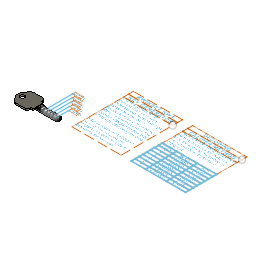
KWIKSET+KW1+KEYGEN (Autodesk Fusion 360 design; units mm, degrees)
Autodesk Fusion 360 part; units mm, degrees
note: some values were not read from the file. Set by a fixed rule: which sketch regions a step uses.
sketch "Sketch1" plane through (0, 0, 0) normal (0, 0, 1) x (1, 0, 0)
  line L0 (0, 0) -> (27.94, 0) construction
  line L1 (0, -4.2418) -> (27.94, -4.2418)
  line L2 (0, 4.2418) -> (27.94, 4.2418)
  line L3 (-3, -6.4) -> (0, -6.4)
  line L4 (0, 6.4) -> (-3, 6.4)
  line L5 (-18.6, 11) -> (-3, 11)
  line L6 (-3, -11) -> (-18.6, -11)
  line L7 (-25, -3.3728) -> (-25, 3.3728)
  line L8 (-18.6, 11) -> (-25, 3.3728)
  line L9 (-25, 11) -> (-33.2141, 11) construction
  line L10 (-18.6, -11) -> (-25, -3.3728)
  line L11 (-18.6, -11) -> (-34.3032, -11) construction
  line L12 (-3, 11) -> (-3, 6.4)
  line L13 (-3, -6.4) -> (-3, -11)
  arc A0 (-3, 8.5) -> (-5.5, 11) centre (-5.5, 8.5) ccw
  arc A1 (-5.5, -11) -> (-3, -8.5) centre (-5.5, -8.5) ccw
  line L14 (27.94, 4.2418) -> (27.94, -4.2418)
  line L15 (23.2107, 4.2418) -> (27.6471, -0.1946)
  line L16 (23.2107, 4.2418) -> (33.0981, 4.2418) construction
  line L17 (0, -0.9017) -> (27.94, -0.9017) construction
  line L18 (25.0141, -4.2418) -> (27.6471, -1.6088)
  line L19 (25.0141, -4.2418) -> (38.1109, -4.2418) construction
  arc A2 (27.6471, -1.6088) -> (27.3724, 0) centre (26.94, -0.9017) ccw
  line L20 (0, 4.2418) -> (0, 6.4)
  line L21 (0, -6.4) -> (0, -4.2418)
  dimension "d6" = 27.94
  dimension "d7" = 4.2418
  dimension "d8" = -4.2418
  dimension "d10" = 6.4
  dimension "d11" = 6.4
  dimension "d13" = 3
  dimension "d14" = 11
  dimension "d15" = 11
  dimension "d17" = 50
  dimension "d19" = 50
  dimension "d21" = 6.4
  dimension "d23" = 5
  dimension "d24" = 5
  dimension "d25" = 22
  dimension "d26" = 7.6272
  dimension "d27" = 7.6272
  dimension "d29" = 45
  dimension "d30" = 3.3401
  dimension "d31" = 2
  dimension "d32" = 45
  constraint coincident L0.start origin
  constraint horizontal L0
  constraint horizontal L3
  constraint vertical L21
  constraint horizontal L4
  constraint coincident L0.start L21
  constraint horizontal L5
  constraint vertical L12
  constraint horizontal L6
  constraint vertical L7
  constraint horizontal L9
  constraint horizontal L11
  constraint tangent L5 A0
  constraint tangent L12 A0
  constraint tangent L6 A1
  constraint tangent L12 A1
  constraint collinear L12 L13
  constraint coincident L5 A0.end
  constraint coincident L12 A0.start
  constraint coincident L13 A1.end
  constraint coincident L6 A1.start
  constraint perpendicular L1 L14
  constraint horizontal L16
  constraint coincident L2 L15.start
  constraint coincident L17.start L21
  constraint coincident L14 L17.end
  constraint perpendicular L14 L17
  constraint coincident L17 A2.centre
  constraint tangent L14 A2
  constraint horizontal L19
  constraint coincident L1 L18.start
  constraint coincident L0.end L14
  constraint tangent L18 A2
  constraint tangent L15 A2
  constraint coincident L0 A2.end
  constraint coincident A2 L15.end
  constraint collinear L20 L21
  measures "d6" distance of L0.start L0.end
  measures "d10" distance of L0 L4
  measures "d11" distance of L0 L3
  measures "d13" distance of L12 L21
  measures "d14" distance of L0 L5
  measures "d15" distance of L0 L6
  measures "d17" angle of L8 L9
  measures "d19" angle of L10 L11
  measures "d21" distance of L9.start L5.start
  measures "d23" diameter of A0
  measures "d24" diameter of A1
  measures "d25" distance of L7 L12
  measures "d26" vertical distance of L5.start L7.end
  measures "d27" vertical distance of L6.end L7.start
  measures "d29" angle of L15 L16
  measures "d30" distance of L1 L17
  measures "d31" diameter of A2
  measures "d32" angle of L18 L19
extrude "Extrude1" add sketch "Sketch1" along normal blind 2 contours L1 L2 L3 L4 L5 L6 L7 L8 L10 L12 L13 A0 A1 L15 L18 A2 L20 L21
fillet "Fillet1" radius 1 2 edges at (0, -6.4, 1) (0, 6.4, 1)
fillet "Fillet1" radius 4 4 edges at (-18.6, -11, 1) (-25, -3.3728, 1) (-25, 3.3728, 1) (-18.6, 11, 1)
sketch "Sketch2" plane through (0, 0, 2) normal (0, 0, 1) x (-1, 0, 0)
  line L0 (3, 6.4) -> (1, 6.4)
  line L1 (0, 5.4) -> (0, 4.2418)
  line L2 (0, 4.2418) -> (-25.0141, 4.2418)
  line L3 (-25.0141, 4.2418) -> (-27.6471, 1.6088)
  arc A0 (-27.6471, 1.6088) -> (-27.6471, 0.1946) centre (-26.94, 0.9017) ccw
  line L4 (-27.6471, 0.1946) -> (-23.2107, -4.2418)
  line L5 (-23.2107, -4.2418) -> (0, -4.2418)
  line L6 (0, -4.2418) -> (0, -5.4)
  line L7 (1, -6.4) -> (3, -6.4)
  line L8 (3, -6.4) -> (3, -8.5)
  arc A1 (3, -8.5) -> (5.5, -11) centre (5.5, -8.5) ccw
  line L9 (5.5, -11) -> (16.7348, -11)
  line L10 (19.7989, -9.5712) -> (24.0642, -4.488)
  line L11 (25, -1.9169) -> (25, 1.9169)
  line L12 (24.0642, 4.488) -> (19.7989, 9.5712)
  line L13 (16.7348, 11) -> (5.5, 11)
  arc A2 (5.5, 11) -> (3, 8.5) centre (5.5, 8.5) ccw
  line L14 (3, 8.5) -> (3, 6.4)
  line L15 (0, 4.2418) -> (0, -4.2418) construction
  line L16 (-6.2738, -4.2418) -> (-6.2738, 4.2418) construction
  line L17 (-10.0838, -4.2418) -> (-10.0838, 4.2418) construction
  line L18 (-13.8938, -4.2418) -> (-13.8938, 4.2418) construction
  line L19 (-17.7038, -4.2418) -> (-17.7038, 4.2418) construction
  line L20 (-21.5138, -4.2418) -> (-21.5138, 4.2418) construction
  line L21 (-5.207, -4.2418) -> (-5.207, 4.2418) construction
  line L22 (-7.3406, -4.2418) -> (-7.3406, 4.2418) construction
  line L23 (-9.017, -4.2418) -> (-9.017, 4.2418) construction
  line L24 (-11.1506, -4.2418) -> (-11.1506, 4.2418) construction
  line L25 (-12.827, -4.2418) -> (-12.827, 4.2418) construction
  line L26 (-14.9606, -4.2418) -> (-14.9606, 4.2418) construction
  line L27 (-16.637, -4.2418) -> (-16.637, 4.2418) construction
  line L28 (-18.7706, -4.2418) -> (-18.7706, 4.2418) construction
  line L29 (-20.447, -4.2418) -> (-20.447, 4.2418) construction
  line L30 (-22.5806, -4.2418) -> (-22.5806, 4.2418) construction
  line L31 (-5.207, -3.5306) -> (-7.3406, -3.5306)
  line L32 (-9.017, -1.778) -> (-11.1506, -1.778)
  line L33 (-12.827, -2.9464) -> (-14.9606, -2.9464)
  line L34 (-16.637, -3.5306) -> (-18.7706, -3.5306)
  line L35 (-20.447, -1.778) -> (-22.5806, -1.778)
  line L36 (-5.207, -3.5306) -> (-0.9644, -7.7732)
  line L37 (-5.207, -3.5306) -> (0.793, -3.5306) construction
  line L38 (-7.3406, -3.5306) -> (-11.5832, -7.7732)
  line L39 (-7.3406, -3.5306) -> (-13.3406, -3.5306) construction
  line L40 (-9.017, -1.778) -> (-4.7744, -6.0206)
  line L41 (-9.017, -1.778) -> (-3.017, -1.778) construction
  line L42 (-11.1506, -1.778) -> (-15.3932, -6.0206)
  line L43 (-11.1506, -1.778) -> (-17.1506, -1.778) construction
  line L44 (-12.827, -2.9464) -> (-8.5844, -7.189)
  line L45 (-12.827, -2.9464) -> (-6.827, -2.9464) construction
  line L46 (-14.9606, -2.9464) -> (-19.2032, -7.189)
  line L47 (-14.9606, -2.9464) -> (-20.9606, -2.9464) construction
  line L48 (-16.637, -3.5306) -> (-12.3944, -7.7732)
  line L49 (-16.637, -3.5306) -> (-10.637, -3.5306) construction
  line L50 (-18.7706, -3.5306) -> (-23.0132, -7.7732)
  line L51 (-18.7706, -3.5306) -> (-24.7706, -3.5306) construction
  line L52 (-20.447, -1.778) -> (-16.2044, -6.0206)
  line L53 (-20.447, -1.778) -> (-14.447, -1.778) construction
  line L54 (-22.5806, -1.778) -> (-26.8232, -6.0206)
  line L55 (-22.5806, -1.778) -> (-28.5806, -1.778) construction
  line L56 (0, 0) -> (25, 0) construction
  circle A3 centre (19.5, 0) radius 2.75
  arc A4 (0, -5.4) -> (1, -6.4) centre (1, -5.4) ccw
  arc A5 (1, 6.4) -> (0, 5.4) centre (1, 5.4) ccw
  arc A6 (16.7348, -11) -> (19.7989, -9.5712) centre (16.7348, -7) ccw
  arc A7 (24.0642, -4.488) -> (25, -1.9169) centre (21, -1.9169) ccw
  arc A8 (25, 1.9169) -> (24.0642, 4.488) centre (21, 1.9169) ccw
  arc A9 (19.7989, 9.5712) -> (16.7348, 11) centre (16.7348, 7) ccw
  dimension "d35" = 6.2738
  dimension "d36" = 10.0838
  dimension "d37" = 13.8938
  dimension "d38" = 17.7038
  dimension "d39" = 21.5138
  dimension "d40" = 1.0668
  dimension "d41" = -1.0668
  dimension "d42" = 1.0668
  dimension "d43" = -1.0668
  dimension "d44" = 1.0668
  dimension "d45" = -1.0668
  dimension "d46" = 1.0668
  dimension "d47" = -1.0668
  dimension "d48" = 1.0668
  dimension "d49" = -1.0668
  dimension "d51" = 6.0198
  dimension "d53" = 7.1882
  dimension "d54" = 7.7724
  dimension "d55" = 6.0198
  dimension "d56" = 45
  dimension "d57" = 6
  dimension "d58" = 45
  dimension "d59" = 6
  dimension "d60" = 45
  dimension "d61" = 6
  dimension "d62" = 45
  dimension "d63" = 6
  dimension "d64" = 45
  dimension "d65" = 6
  dimension "d66" = 45
  dimension "d67" = 6
  dimension "d68" = 45
  dimension "d69" = 6
  dimension "d70" = 45
  dimension "d71" = 6
  dimension "d72" = 45
  dimension "d73" = 6
  dimension "d74" = 45
  dimension "d75" = 6
  dimension "d76" = 5.5
  dimension "d77" = 5.5
  dimension "d123" = 7.7724
  constraint coincident L1.end L2.start
  constraint coincident L5.end L6.start
  constraint coincident L5 L16.start
  constraint coincident L2 L16.end
  constraint perpendicular L2 L16
  constraint coincident L5 L17.start
  constraint coincident L2 L17.end
  constraint perpendicular L2 L17
  constraint coincident L5 L18.start
  constraint coincident L2 L18.end
  constraint perpendicular L2 L18
  constraint coincident L5 L19.start
  constraint coincident L2 L19.end
  constraint perpendicular L2 L19
  constraint coincident L5 L20.start
  constraint coincident L2 L20.end
  constraint perpendicular L2 L20
  constraint coincident L21 L31.start
  constraint coincident L22 L31.end
  constraint perpendicular L22 L31
  constraint coincident L23 L32.start
  constraint coincident L24 L32.end
  constraint perpendicular L24 L32
  constraint coincident L25 L33.start
  constraint coincident L26 L33.end
  constraint perpendicular L26 L33
  constraint coincident L27 L34.start
  constraint coincident L28 L34.end
  constraint perpendicular L28 L34
  constraint coincident L29 L35.start
  constraint coincident L30 L35.end
  constraint perpendicular L30 L35
  constraint horizontal L37
  constraint horizontal L39
  constraint horizontal L41
  constraint horizontal L43
  constraint horizontal L45
  constraint horizontal L47
  constraint horizontal L49
  constraint horizontal L51
  constraint horizontal L53
  constraint horizontal L55
  constraint coincident L56.start origin
  constraint perpendicular L15 L56
  constraint coincident L11 L56.end
  constraint coincident L56 A3.centre
  measures "d35" distance of L15 L16
  measures "d36" distance of L15 L17
  measures "d37" distance of L15 L18
  measures "d38" distance of L15 L19
  measures "d39" distance of L15 L20
  measures "d51" distance of L2 L32
  measures "d53" distance of L2 L33
  measures "d54" distance of L2 L34
  measures "d55" distance of L2 L35
  measures "d56" angle of L36 L37
  measures "d57" distance of L31.start L36.end
  measures "d58" angle of L38 L39
  measures "d59" distance of L31.end L38.end
  measures "d60" angle of L40 L41
  measures "d61" distance of L32.start L40.end
  measures "d62" angle of L42 L43
  measures "d63" distance of L32.end L42.end
  measures "d64" angle of L44 L45
  measures "d65" distance of L33.start L44.end
  measures "d66" angle of L46 L47
  measures "d67" distance of L33.end L46.end
  measures "d68" angle of L48 L49
  measures "d69" distance of L34.start L48.end
  measures "d70" angle of L50 L51
  measures "d71" distance of L34.end L50.end
  measures "d72" angle of L52 L53
  measures "d73" distance of L35.start L52.end
  measures "d74" angle of L54 L55
  measures "d75" distance of L35.end L54.end
  measures "d76" diameter of A3
  measures "d77" distance of L11 A3.centre
  measures "d123" distance of L2 L31
extrude "Extrude2" cut sketch "Sketch2" against normal blind 2 contours L0 L1 L2 L3 A0 L4 L5 L6 L7 L8 A1 L9 L10 L11 L12 L13 A2 L14 L31 L32 L33 L34 L35 L36 L40 L42 L44 L46 L48 L52 L54 A4 A5 A6 A7 A8 A9 keep common part
sketch "Sketch3" plane through (0, 0, 0) normal (1, 0, 0) x (0, 1, 0)
  line L0 (4.2418, 0) -> (4.2418, 2)
  line L1 (-4.2418, 0) -> (-4.2418, 2)
  line L2 (-4.2418, 2) -> (4.2418, 2)
  line L3 (-4.2418, 0) -> (4.2418, 0)
  line L4 (-3.5418, 0.75) -> (-3.5418, 2)
  line L5 (-2.1418, 2) -> (-2.1418, 0.75)
  line L6 (0.6082, 2) -> (0.6082, 1.49)
  line L7 (-1.3918, 1.25) -> (-1.3918, 0)
  line L8 (0.0082, 1.25) -> (0.0082, 0)
  line L9 (-3.5418, 0.75) -> (-2.1418, 0.75)
  line L10 (-1.3918, 1.25) -> (0.0082, 1.25)
  line L11 (0.9582, 1.14) -> (4.2418, 1.14)
  line L12 (0.6082, 1.49) -> (0.9582, 1.14)
  line L13 (0.6082, 1.49) -> (1.6082, 1.49) construction
  line L14 (-1.3918, 0.9) -> (-1.0418, 1.25)
  line L15 (-1.3918, 0.9) -> (-0.3918, 0.9) construction
  line L16 (0.0082, 0.9) -> (-0.3418, 1.25)
  line L17 (0.0082, 0.9) -> (-0.9918, 0.9) construction
  line L18 (-3.5418, 1.1) -> (-2.5418, 1.1) construction
  line L19 (-2.1418, 1.1) -> (-3.1418, 1.1) construction
  line L20 (-3.5418, 1.1) -> (-3.1918, 0.75)
  line L21 (-2.8418, 0.4) -> (-2.8347, 0.3929) construction
  line L22 (-2.1418, 1.1) -> (-2.4918, 0.75)
  line L23 (-2.8418, 0.4) -> (-2.8489, 0.3929) construction
  arc A0 (-1.9418, 2) -> (-2.1418, 1.8) centre (-1.9418, 1.8) ccw
  arc A1 (0.6082, 1.8) -> (0.4082, 2) centre (0.4082, 1.8) ccw
  arc A2 (0.0082, 0.2) -> (0.2082, 0) centre (0.2082, 0.2) ccw
  arc A3 (-1.5918, 0) -> (-1.3918, 0.2) centre (-1.5918, 0.2) ccw
  point P0 (-4.2418, 0)
  point P1 (-4.2418, 2)
  dimension "d84" = 0.7
  dimension "d85" = 1.4
  dimension "d86" = 2.75
  dimension "d87" = 2.85
  dimension "d88" = 1.4
  dimension "d90" = 0.75
  dimension "d92" = 1.25
  dimension "d93" = 0.86
  dimension "d96" = 45
  dimension "d99" = 45
  dimension "d101" = 45
  dimension "d103" = 0.35
  dimension "d104" = 0.35
  dimension "d105" = 45
  dimension "d106" = 1
  dimension "d107" = 45
  dimension "d108" = 1
  dimension "d109" = 0.35
  dimension "d110" = 0.35
  dimension "d111" = 0.35
  dimension "d112" = 0.4
  dimension "d113" = 0.4
  dimension "d114" = 0.4
  dimension "d115" = 0.4
  constraint coincident P1 L1.end
  constraint coincident L0.end L2.end
  constraint coincident P0 L1.start
  constraint coincident L0.start L3.end
  constraint coincident L2 L4.end
  constraint perpendicular L2 L4
  constraint coincident L2 L5.start
  constraint perpendicular L3 L5
  constraint coincident L2 L6.start
  constraint perpendicular L3 L6
  constraint coincident L3 L7.end
  constraint perpendicular L3 L7
  constraint coincident L3 L8.end
  constraint perpendicular L3 L8
  constraint coincident L0 L11.end
  constraint perpendicular L0 L9
  constraint horizontal L13
  constraint horizontal L15
  constraint coincident L7 L14.start
  constraint horizontal L17
  constraint coincident L8 L16.start
  constraint coincident L10 L16.end
  constraint coincident L10 L14.end
  constraint horizontal L18
  constraint coincident L4 L18.start
  constraint horizontal L19
  constraint coincident L5 L19.start
  constraint coincident L9 L20.end
  constraint coincident L21.start L22
  constraint collinear L20 L21
  constraint coincident L9 L22.end
  constraint collinear L22 L23
  constraint tangent L3 A3
  constraint tangent L7 A3
  constraint tangent L8 A2
  constraint tangent L3 A2
  constraint tangent L2 A1
  constraint tangent L6 A1
  constraint tangent L2 A0
  constraint tangent L5 A0
  constraint coincident L5 A0.end
  constraint coincident L2 A0.start
  constraint coincident L2 A1.end
  constraint coincident L6 A1.start
  constraint coincident L3 A2.end
  constraint coincident L8 A2.start
  constraint coincident L7 A3.end
  constraint coincident L3 A3.start
  measures "d84" distance of L1 L4
  measures "d85" distance of L4 L5
  measures "d86" distance of L5 L6
  measures "d87" distance of L1 L7
  measures "d88" distance of L7 L8
  measures "d90" distance of L3 L9
  measures "d92" distance of L3 L10
  measures "d93" distance of L2 L11
  measures "d96" angle of L12 L13
  measures "d99" angle of L14 L15
  measures "d101" angle of L16 L17
  measures "d103" distance of L7.start L14.start
  measures "d104" distance of L8.start L16.start
  measures "d105" angle of L18 L20
  measures "d106" distance of L18.start L21.end
  measures "d107" angle of L19 L22
  measures "d108" distance of L19.start L23.end
  measures "d109" distance of L9 L18.start
  measures "d110" distance of L5.end L19.start
  measures "d111" vertical distance of L6.end L11.start
  measures "d112" diameter of A0
  measures "d113" diameter of A1
  measures "d114" diameter of A3
  measures "d115" diameter of A2
extrude "Extrude3" cut sketch "Sketch3" along normal blind 30 contours L0 L2 L6 L11 L12 | L3 L8 A2 | L3 L7 L8 L10 L14 L16 | L2 L6 A1 | L3 L7 A3 | L2 L5 A0 | L2 L4 L5 L9 L20 L22
sketch "Sketch4" plane through (0, 0, 0) normal (0, 0, 1) x (1, 0, 0)
  line L0 (6.2738, 0) -> (6.2738, 35)
  line L1 (10.0838, 0) -> (10.0838, 30)
  line L2 (13.8938, 0) -> (13.8938, 25)
  line L3 (17.7038, 0) -> (17.7038, 20)
  line L4 (21.5138, 0) -> (21.5138, 15)
  line L5 (6.2738, 35) -> (16.2738, 35) construction
  line L6 (16.2738, 35) -> (16.2738, 39) construction
  line L7 (16.2738, 39) -> (6.2738, 39) construction
  line L8 (6.2738, 39) -> (6.2738, 35) construction
  line L9 (10.0838, 30) -> (20.0838, 30) construction
  line L10 (20.0838, 30) -> (20.0838, 34) construction
  line L11 (20.0838, 34) -> (10.0838, 34) construction
  line L12 (10.0838, 34) -> (10.0838, 30) construction
  line L13 (13.8938, 25) -> (23.8938, 25) construction
  line L14 (23.8938, 25) -> (23.8938, 29) construction
  line L15 (23.8938, 29) -> (13.8938, 29) construction
  line L16 (13.8938, 29) -> (13.8938, 25) construction
  line L17 (17.7038, 20) -> (27.7038, 20) construction
  line L18 (27.7038, 20) -> (27.7038, 24) construction
  line L19 (27.7038, 24) -> (17.7038, 24) construction
  line L20 (17.7038, 24) -> (17.7038, 20) construction
  line L21 (21.5138, 15) -> (31.5138, 15) construction
  line L22 (31.5138, 15) -> (31.5138, 19) construction
  line L23 (31.5138, 19) -> (21.5138, 19) construction
  line L24 (21.5138, 19) -> (21.5138, 15) construction
  line L25 (40.8004, 0.0886) -> (100.8004, 0.0886) construction
  line L26 (100.8004, 0.0886) -> (100.8004, 75.0886) construction
  line L27 (100.8004, 75.0886) -> (40.8004, 75.0886) construction
  line L28 (40.8004, 75.0886) -> (40.8004, 0.0886) construction
  line L29 (100.8004, 69.0886) -> (40.8004, 69.0886) construction
  line L30 (40.8004, 69.0886) -> (100.8004, 69.0886) construction
  line L31 (100.8004, 69.0886) -> (100.8004, 75.0886) construction
  line L32 (100.8004, 75.0886) -> (40.8004, 75.0886) construction
  line L33 (40.8004, 75.0886) -> (40.8004, 69.0886) construction
  line L34 (100.8004, 63.0886) -> (40.8004, 63.0886) construction
  line L35 (40.8004, 63.0886) -> (100.8004, 63.0886) construction
  line L36 (100.8004, 63.0886) -> (100.8004, 69.0886) construction
  line L37 (100.8004, 69.0886) -> (40.8004, 69.0886) construction
  line L38 (40.8004, 69.0886) -> (40.8004, 63.0886) construction
  line L39 (40.8004, 0.1102) -> (100.8004, 0.1102) construction
  line L40 (100.8004, 0.1102) -> (100.8004, 63.0886) construction
  line L41 (100.8004, 63.0886) -> (40.8004, 63.0886) construction
  line L42 (40.8004, 63.0886) -> (40.8004, 0.1102) construction
  line L43 (113.1762, 75.0886) -> (179.487, 75.0886) construction
  line L44 (179.487, 75.0886) -> (179.487, 0.0886) construction
  line L45 (179.487, 0.0886) -> (113.1762, 0.0886) construction
  line L46 (113.1762, 0.0886) -> (113.1762, 75.0886) construction
  line L47 (113.1762, 69.0886) -> (179.487, 69.0886) construction
  line L48 (113.1762, 63.0886) -> (179.487, 63.0886) construction
  line L49 (113.1762, 69.0886) -> (179.487, 69.0886) construction
  line L50 (179.487, 69.0886) -> (179.487, 75.0886) construction
  line L51 (179.487, 75.0886) -> (113.1762, 75.0886) construction
  line L52 (113.1762, 75.0886) -> (113.1762, 69.0886) construction
  line L53 (113.1762, 63.0886) -> (179.487, 63.0886) construction
  line L54 (179.487, 63.0886) -> (179.487, 69.0886) construction
  line L55 (179.487, 69.0886) -> (113.1762, 69.0886) construction
  line L56 (113.1762, 69.0886) -> (113.1762, 63.0886) construction
  line L57 (113.1762, 38.0886) -> (179.487, 38.0886) construction
  line L58 (113.1762, 38.0886) -> (179.487, 38.0886) construction
  line L59 (179.487, 38.0886) -> (179.487, 63.0886) construction
  line L60 (179.487, 63.0886) -> (113.1762, 63.0886) construction
  line L61 (113.1762, 63.0886) -> (113.1762, 38.0886) construction
  line L62 (179.487, 4.8386) -> (113.1762, 4.8386) construction
  line L63 (179.487, 9.5886) -> (113.1762, 9.5886) construction
  line L64 (179.487, 14.3386) -> (113.1762, 14.3386) construction
  line L65 (179.487, 19.0886) -> (113.1762, 19.0886) construction
  line L66 (179.487, 23.8386) -> (113.1762, 23.8386) construction
  line L67 (179.487, 28.5886) -> (113.1762, 28.5886) construction
  line L68 (179.487, 33.3386) -> (113.1762, 33.3386) construction
  line L69 (113.1762, 38.0886) -> (179.487, 38.0886)
  line L70 (179.487, 38.0886) -> (179.487, 0.0886)
  line L71 (179.487, 0.0886) -> (113.1762, 0.0886)
  line L72 (113.1762, 0.0886) -> (113.1762, 38.0886)
  line L73 (113.1762, 4.8386) -> (179.487, 4.8386)
  line L74 (179.487, 9.5886) -> (113.1762, 9.5886)
  line L75 (113.1762, 14.3386) -> (179.487, 14.3386)
  line L76 (113.1762, 19.0886) -> (179.487, 19.0886)
  line L77 (113.1762, 23.8386) -> (179.487, 23.8386)
  line L78 (113.1762, 28.5886) -> (179.487, 28.5886)
  line L79 (113.1762, 33.3386) -> (179.487, 33.3386)
  line L80 (130.6528, 38.0886) -> (130.6528, 0.0886)
  line L81 (155.9913, 38.0886) -> (155.9913, 0.0886)
  line L82 (113.1762, 33.3386) -> (130.6528, 33.3386) construction
  line L83 (130.6528, 33.3386) -> (130.6528, 38.0886) construction
  line L84 (130.6528, 38.0886) -> (113.1762, 38.0886) construction
  line L85 (113.1762, 38.0886) -> (113.1762, 33.3386) construction
  line L86 (130.6528, 33.3386) -> (155.9913, 33.3386) construction
  line L87 (155.9913, 33.3386) -> (155.9913, 38.0886) construction
  line L88 (155.9913, 38.0886) -> (130.6528, 38.0886) construction
  line L89 (130.6528, 38.0886) -> (130.6528, 33.3386) construction
  line L90 (155.9913, 33.3386) -> (179.487, 33.3386) construction
  line L91 (179.487, 33.3386) -> (179.487, 38.0886) construction
  line L92 (179.487, 38.0886) -> (155.9913, 38.0886) construction
  line L93 (155.9913, 38.0886) -> (155.9913, 33.3386) construction
  line L94 (113.1762, 28.5886) -> (130.6528, 28.5886) construction
  line L95 (130.6528, 28.5886) -> (130.6528, 33.3386) construction
  line L96 (130.6528, 33.3386) -> (113.1762, 33.3386) construction
  line L97 (113.1762, 33.3386) -> (113.1762, 28.5886) construction
  line L98 (113.1762, 23.8386) -> (130.6528, 23.8386) construction
  line L99 (130.6528, 23.8386) -> (130.6528, 28.5886) construction
  line L100 (130.6528, 28.5886) -> (113.1762, 28.5886) construction
  line L101 (113.1762, 28.5886) -> (113.1762, 23.8386) construction
  line L102 (113.1762, 19.0886) -> (130.6528, 19.0886) construction
  line L103 (130.6528, 19.0886) -> (130.6528, 23.8386) construction
  line L104 (130.6528, 23.8386) -> (113.1762, 23.8386) construction
  line L105 (113.1762, 23.8386) -> (113.1762, 19.0886) construction
  line L106 (113.1762, 14.3386) -> (130.6528, 14.3386) construction
  line L107 (130.6528, 14.3386) -> (130.6528, 19.0886) construction
  line L108 (130.6528, 19.0886) -> (113.1762, 19.0886) construction
  line L109 (113.1762, 19.0886) -> (113.1762, 14.3386) construction
  line L110 (113.1762, 9.5886) -> (130.6528, 9.5886) construction
  line L111 (130.6528, 9.5886) -> (130.6528, 14.3386) construction
  line L112 (130.6528, 14.3386) -> (113.1762, 14.3386) construction
  line L113 (113.1762, 14.3386) -> (113.1762, 9.5886) construction
  line L114 (113.1762, 4.8386) -> (130.6528, 4.8386) construction
  line L115 (130.6528, 4.8386) -> (130.6528, 9.5886) construction
  line L116 (130.6528, 9.5886) -> (113.1762, 9.5886) construction
  line L117 (113.1762, 9.5886) -> (113.1762, 4.8386) construction
  line L118 (113.1762, 0.0886) -> (130.6528, 0.0886) construction
  line L119 (130.6528, 0.0886) -> (130.6528, 4.8386) construction
  line L120 (130.6528, 4.8386) -> (113.1762, 4.8386) construction
  line L121 (113.1762, 4.8386) -> (113.1762, 0.0886) construction
  line L122 (155.9913, 28.5886) -> (179.487, 28.5886) construction
  line L123 (179.487, 28.5886) -> (179.487, 33.3386) construction
  line L124 (179.487, 33.3386) -> (155.9913, 33.3386) construction
  line L125 (155.9913, 33.3386) -> (155.9913, 28.5886) construction
  line L126 (155.9913, 23.8386) -> (179.487, 23.8386) construction
  line L127 (179.487, 23.8386) -> (179.487, 28.5886) construction
  line L128 (179.487, 28.5886) -> (155.9913, 28.5886) construction
  line L129 (155.9913, 28.5886) -> (155.9913, 23.8386) construction
  line L130 (155.9913, 19.0886) -> (179.487, 19.0886) construction
  line L131 (179.487, 19.0886) -> (179.487, 23.8386) construction
  line L132 (179.487, 23.8386) -> (155.9913, 23.8386) construction
  line L133 (155.9913, 23.8386) -> (155.9913, 19.0886) construction
  line L134 (155.9913, 14.3386) -> (179.487, 14.3386) construction
  line L135 (179.487, 14.3386) -> (179.487, 19.0886) construction
  line L136 (179.487, 19.0886) -> (155.9913, 19.0886) construction
  line L137 (155.9913, 19.0886) -> (155.9913, 14.3386) construction
  line L138 (155.9913, 9.5886) -> (179.487, 9.5886) construction
  line L139 (179.487, 9.5886) -> (179.487, 14.3386) construction
  line L140 (179.487, 14.3386) -> (155.9913, 14.3386) construction
  line L141 (155.9913, 14.3386) -> (155.9913, 9.5886) construction
  line L142 (155.9913, 4.8386) -> (179.487, 4.8386) construction
  line L143 (179.487, 4.8386) -> (179.487, 9.5886) construction
  line L144 (179.487, 9.5886) -> (155.9913, 9.5886) construction
  line L145 (155.9913, 9.5886) -> (155.9913, 4.8386) construction
  line L146 (155.9913, 0.0886) -> (179.487, 0.0886) construction
  line L147 (179.487, 0.0886) -> (179.487, 4.8386) construction
  line L148 (179.487, 4.8386) -> (155.9913, 4.8386) construction
  line L149 (155.9913, 4.8386) -> (155.9913, 0.0886) construction
  line L150 (130.6528, 28.5886) -> (155.9913, 28.5886) construction
  line L151 (155.9913, 28.5886) -> (155.9913, 33.3386) construction
  line L152 (155.9913, 33.3386) -> (130.6528, 33.3386) construction
  line L153 (130.6528, 33.3386) -> (130.6528, 28.5886) construction
  line L154 (130.6528, 23.8386) -> (155.9913, 23.8386) construction
  line L155 (155.9913, 23.8386) -> (155.9913, 28.5886) construction
  line L156 (155.9913, 28.5886) -> (130.6528, 28.5886) construction
  line L157 (130.6528, 28.5886) -> (130.6528, 23.8386) construction
  line L158 (130.6528, 19.0886) -> (155.9913, 19.0886) construction
  line L159 (155.9913, 19.0886) -> (155.9913, 23.8386) construction
  line L160 (155.9913, 23.8386) -> (130.6528, 23.8386) construction
  line L161 (130.6528, 23.8386) -> (130.6528, 19.0886) construction
  line L162 (130.6528, 14.3386) -> (155.9913, 14.3386) construction
  line L163 (155.9913, 14.3386) -> (155.9913, 19.0886) construction
  line L164 (155.9913, 19.0886) -> (130.6528, 19.0886) construction
  line L165 (130.6528, 19.0886) -> (130.6528, 14.3386) construction
  line L166 (130.6528, 9.5886) -> (155.9913, 9.5886) construction
  line L167 (155.9913, 9.5886) -> (155.9913, 14.3386) construction
  line L168 (155.9913, 14.3386) -> (130.6528, 14.3386) construction
  line L169 (130.6528, 14.3386) -> (130.6528, 9.5886) construction
  line L170 (130.6528, 4.8386) -> (155.9913, 4.8386) construction
  line L171 (155.9913, 4.8386) -> (155.9913, 9.5886) construction
  line L172 (155.9913, 9.5886) -> (130.6528, 9.5886) construction
  line L173 (130.6528, 9.5886) -> (130.6528, 4.8386) construction
  line L174 (130.6528, 0.0886) -> (155.9913, 0.0886) construction
  line L175 (155.9913, 0.0886) -> (155.9913, 4.8386) construction
  line L176 (155.9913, 4.8386) -> (130.6528, 4.8386) construction
  line L177 (130.6528, 4.8386) -> (130.6528, 0.0886) construction
  dimension "d125" = 35
  dimension "d126" = 30
  dimension "d127" = 25
  dimension "d128" = 20
  dimension "d129" = 15
  dimension "d140" = 3
  dimension "d141" = 3
  dimension "d142" = 3
  dimension "d143" = 3
  dimension "d144" = 3
  dimension "d145" = 60
  dimension "d146" = 75
  dimension "d147" = -6
  dimension "d148" = 4
  dimension "d149" = -12
  dimension "d150" = 4
  dimension "d151" = 3
  dimension "d152" = 6
  dimension "d153" = 12
  dimension "d154" = 4
  dimension "d155" = 4
  dimension "d156" = 25
  dimension "d157" = 3
  dimension "d158" = 75
  dimension "d159" = 75
  dimension "d163" = 0
  dimension "d164" = 4.75
  dimension "d165" = 3
  dimension "d166" = 3
  dimension "d167" = 3
  dimension "d168" = 3
  dimension "d169" = 3
  dimension "d170" = 3
  dimension "d171" = 3
  dimension "d172" = 3
  dimension "d173" = 3
  dimension "d174" = 3
  dimension "d175" = 3
  dimension "d176" = 3
  dimension "d177" = 3
  dimension "d178" = 3
  dimension "d179" = 3
  dimension "d180" = 3
  dimension "d181" = 3
  dimension "d182" = 3
  dimension "d183" = 3
  dimension "d184" = 3
  dimension "d185" = 3
  dimension "d186" = 3
  dimension "d187" = 3
  dimension "d188" = 3
  constraint coincident L0.end
  constraint coincident L1.end
  constraint coincident L2.end
  constraint coincident L3.end
  constraint coincident L4.end
  constraint horizontal L25
  constraint vertical L26
  constraint horizontal L27
  constraint vertical L28
  constraint coincident L26.end
  constraint coincident L29.end
  constraint coincident L29.start
  constraint coincident L34.end
  constraint coincident L26
  constraint horizontal L43
  constraint vertical L44
  constraint horizontal L45
  constraint vertical L46
  constraint coincident L43.end
  constraint coincident L47.start
  constraint coincident L48.end
  constraint coincident L46 L57.start
  constraint coincident L44 L57.end
  constraint perpendicular L44 L57
  constraint coincident L57.end
  constraint coincident L48.start
  constraint horizontal L69
  constraint vertical L70
  constraint horizontal L71
  constraint vertical L72
  constraint coincident L57.start
  constraint coincident L57 L80.start
  constraint coincident L45 L80.end
  constraint perpendicular L45 L80
  constraint coincident L69 L81.start
  constraint coincident L45 L81.end
  constraint perpendicular L45 L81
  constraint coincident L80.start
  constraint coincident L68.end
  constraint coincident L81
  constraint coincident L79
  constraint coincident L68.start
  constraint coincident L81.start
  constraint coincident L80
  constraint coincident L78
  constraint coincident L66
  constraint coincident L67.end
  constraint midpoint L80
  constraint coincident L66.end
  constraint coincident L75
  constraint coincident L63
  constraint coincident L73
  constraint coincident L80.end
  constraint coincident L67.start
  constraint coincident L66.start
  constraint coincident L65.start
  constraint coincident L64.start
  constraint coincident L63.start
  constraint coincident L62.start
  constraint coincident L44.end
  constraint coincident L81.end
  measures "d125" distance of L0.start L0.end
  measures "d126" distance of L1.start L1.end
  measures "d127" distance of L2.start L2.end
  measures "d128" distance of L3.start L3.end
  measures "d129" distance of L4.start L4.end
  measures "d145" distance of L25.start L25.end
  measures "d146" distance of L25.start L27.end
  measures "d156" distance of L48 L57
  measures "d158" distance of L45 L51
  measures "d159" distance of L25 L51
equation "d6 = ( 1.1 * 25.4 ) * 1 mm"
equation "d7 = ( 0.334 * 12.7 ) * 1 mm"
equation "d8 = ( 0.334 * -12.7 ) * 1 mm"
equation "d30 = ( ( 0.334 - 0.2025 ) * 25.4 ) * 1 mm"
equation "d35 = ( 0.247 * 25.4 ) * 1 mm"
equation "d36 = ( 0.397 * 25.4 ) * 1 mm"
equation "d37 = ( 0.547 * 25.4 ) * 1 mm"
equation "d38 = ( 0.697 * 25.4 ) * 1 mm"
equation "d39 = ( 0.847 * 25.4 ) * 1 mm"
equation "d40 = ( 0.042 * 25.4 ) * 1 mm"
equation "d41 = ( 0.042 * -25.4 ) * 1 mm"
equation "d42 = ( 0.042 * 25.4 ) * 1 mm"
equation "d43 = ( 0.042 * -25.4 ) * 1 mm"
equation "d44 = ( 0.042 * 25.4 ) * 1 mm"
equation "d45 = ( 0.042 * -25.4 ) * 1 mm"
equation "d46 = ( 0.042 * 25.4 ) * 1 mm"
equation "d47 = ( 0.042 * -25.4 ) * 1 mm"
equation "d48 = ( 0.042 * 25.4 ) * 1 mm"
equation "d49 = ( 0.042 * -25.4 ) * 1 mm"
equation "d51 = ( ( 0.168 + ( 0.023 * ( 8 - CUT_2 ) ) ) * 25.4 ) * 1 mm"
equation "d53 = ( ( 0.168 + ( 0.023 * ( 8 - CUT_3 ) ) ) * 25.4 ) * 1 mm"
equation "d54 = ( ( 0.168 + ( 0.023 * ( 8 - CUT_4 ) ) ) * 25.4 ) * 1 mm"
equation "d55 = ( ( 0.168 + ( 0.023 * ( 8 - CUT_5 ) ) ) * 25.4 ) * 1 mm"
equation "CUT_1 = floor(KEYCODE / 10000)" comment "DON'T CHANGE THIS"
equation "CUT_2 = floor(( KEYCODE - ( floor(KEYCODE / 10000) * 10000 ) ) / 1000)" comment "DON'T CHANGE THIS"
equation "CUT_3 = floor(( KEYCODE - ( floor(KEYCODE / 1000) * 1000 ) ) / 100)" comment "DON'T CHANGE THIS"
equation "CUT_4 = floor(( KEYCODE - ( floor(KEYCODE / 100) * 100 ) ) / 10)" comment "DON'T CHANGE THIS"
equation "CUT_5 = floor(( KEYCODE - ( floor(KEYCODE / 10) * 10 ) ) / 1)" comment "DON'T CHANGE THIS"
equation "d123 = ( ( 0.168 + ( 0.023 * ( 8 - CUT_1 ) ) ) * 25.4 ) * 1 mm"
equation "KEYCODE = 25325" comment "ENTER THE KEYCODE HERE"
